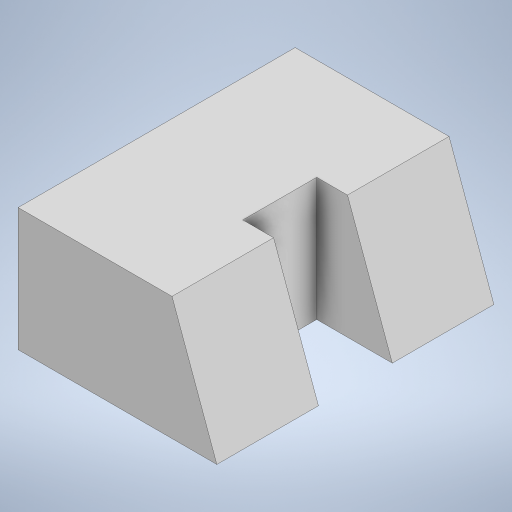
# Autodesk Inventor part: 4-3拔模2
Saved by Autodesk Inventor 2024.2 (Build 282272000, 272)
## iProperties
Created: 2024-03-28
Part Number: 4-3拔模2
Material: 一般
Document SubType Name: Modeling
Designer: User
Density: 1 g/cm^3
Appearance: 預設
Author: User
Autodesk Inventor part; units mm, degrees
ref_plane "YZ Plane" through (0, 0, 0) normal (1, 0, 0) x (0, 1, 0)
ref_plane "XZ Plane" through (0, 0, 0) normal (0, 1, 0) x (-1, 0, 0)
ref_plane "XY Plane" through (0, 0, 0) normal (0, 0, 1) x (1, 0, 0)
sketch "草圖1" plane through (0, 0, 0) normal (0, 0, 1) x (1, 0, 0)
  line L0 (0, 0) -> (25, 0)
  line L1 (25, 0) -> (25, 20)
  line L2 (25, 20) -> (0, 20)
  line L3 (0, 20) -> (0, 0)
  dimension "d0" = 25
  dimension "d1" = 20
  constraints: 8 end point, 2 parallel, 1 horizontal, 1 perpendicular
  measures "d0" distance of L2.end L1.end
  measures "d1" distance of L1.end L0.end
extrude "擠出1" add sketch "草圖1" along normal blind 45
sketch "草圖2" plane through (0, 20, 0) normal (0, 1, 0) x (1, 0, 0)
  line L0 (25, -22.5) -> (25, -16.5)
  line L1 (25, -22.5) -> (25, -28.5)
  line L2 (25, -28.5) -> (20, -28.5)
  line L3 (20, -28.5) -> (20, -16.5)
  line L4 (20, -16.5) -> (25, -16.5)
  line L5 (25, -16.5) -> (25, -28.5)
  point P0 (0, 0)
  point P1 (25, 0)
  dimension "d4" = 22.5
  dimension "d5" = 6
  dimension "d6" = 6
  dimension "d7" = 5
  dimension "d8" = 12
  constraints: 12 end point, 1 collinear
  measures "d4" distance of point (25, 0) L0.start
  measures "d5" distance of L0.end L0.start
  measures "d6" distance of L0.start L1.end
  measures "d7" distance of L1.end L2.end
  measures "d8" distance of L2.end L3.end
extrude "擠出2" cut sketch "草圖2" against normal blind 20
draft "面拔模1" angle 20 pull direction (0, 1, 0) fixed plane through (6.6667, 20, 24.5) normal (0, 1, 0) faces at (25, 6.6667, 34) (25, 6.6667, 5.5)
